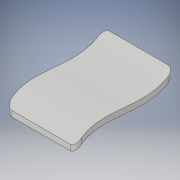
# Autodesk Inventor part: Case Top
Saved by Autodesk Inventor 2019 (Build 230136000, 136)
## iProperties
Created: 2022-04-25
Part Number: Case Top
Material: Generic
Document SubType Name: Modeling
Designer: Loxei
Density: 1 g/cm^3
Appearance: Default
Author: Loxei
Autodesk Inventor part; units mm, degrees
ref_plane "YZ Plane" through (0, 0, 0) normal (1, 0, 0) x (0, 1, 0)
ref_plane "XZ Plane" through (0, 0, 0) normal (0, 1, 0) x (-1, 0, 0)
ref_plane "XY Plane" through (0, 0, 0) normal (0, 0, 1) x (1, 0, 0)
sketch "Sketch2" plane through (0, 0, 0) normal (1, 0, 0) x (0, 1, 0)
  line L0 (-1.8268, 35) -> (17.968, 20.835) construction
  line L1 (17.968, 20.835) -> (-5.8268, -16.2285) construction
  line L2 (-5.8268, -16.2285) -> (12.551, -35) construction
  spline S0 degree 3 poles (-1.8268, 35) (17.968, 20.835) (-5.8268, -16.2285) (12.551, -35) knots 1 1 1 1 2 2 2 2
  line L3 (43.3052, 0) -> (-43.3052, 0) construction
  line L4 (0, 65.4619) -> (0, -65.4619) construction
  line L5 (12.551, -35) -> (8.551, -35)
  line L6 (-5.8268, 35) -> (13.8832, 21.2522) construction
  line L7 (13.8832, 21.2522) -> (-10.0462, -16.0043) construction
  line L8 (-10.0462, -16.0043) -> (8.551, -35) construction
  spline S1 degree 3 poles (-5.8268, 35) (13.8832, 21.2522) (-10.0462, -16.0043) (8.551, -35) knots 1 1 1 1 2 2 2 2
  line L9 (-1.8268, 35) -> (-5.8268, 35)
  point P0 (0, 0)
  point P1 (0, 0)
  point P2 (0, 0)
  dimension "d0" = 70
  dimension "d1" = 35
  dimension "d3" = 4
  dimension "d4" = 4
  constraints: 8 end point, 3 horizontal, 3 midpoint, 2 symmetric about line, 1 coincident, 1 perpendicular, 1 vertical, 6 other
  measures "d0" vertical distance of L0.start L2.end
  measures "d1" vertical distance of point (0, 0) L2.end
  measures "d3" distance of L2.end L5.end
  measures "d4" distance of L0.start L6.start
extrude "Extrusion1" add sketch "Sketch2" along normal blind 50
fillet "Fillet1" radius 4 4 edges at (50, -3.8268, 35) (0, -3.8268, 35) (50, 10.551, -35) (0, 10.551, -35)
equation "\"d4\" = d3"
body "Solid1"
